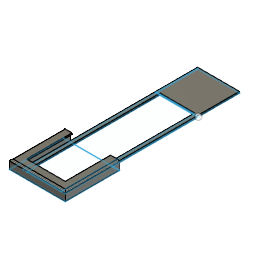
assembled (Autodesk Fusion 360 archive; units mm, degrees)
design "Dongle v3"
part number: 2026-08-27-20-51-44-399
Autodesk Fusion 360 part; units mm, degrees
sketch "snippy-Edge_Cuts" plane through (0, 0, 0) normal (0, 1, 0) x (1, 0, 0)
  line L0 (73.4, -145) -> (85.6, -145)
  line L1 (85.6, -145) -> (85.6, -157)
  line L2 (85.6, -157) -> (73.4, -157)
  line L3 (73.4, -157) -> (73.4, -145)
  line L4 (73.4, -145) -> (73.4, -157)
  line L5 (73.4, -157) -> (85.6, -157)
  line L6 (85.6, -157) -> (85.6, -195.7)
  line L7 (85.6, -195.7) -> (73.4, -195.7)
  line L8 (73.4, -195.7) -> (73.4, -157)
  line L9 (87.6, -182) -> (87.6, -197.7)
  line L10 (87.6, -197.7) -> (71.4, -197.7)
  line L11 (71.4, -197.7) -> (71.4, -182)
  line L12 (73.4, -157) -> (85.6, -157)
  line L13 (84.5, -157) -> (74.5, -157)
  line L14 (74.5, -157) -> (74.5, -195.7)
  line L15 (74.5, -195.7) -> (84.5, -195.7)
  line L16 (84.5, -195.7) -> (84.5, -157)
  line L17 (85.6, -157) -> (85.6, -182)
  line L18 (85.6, -182) -> (87.6, -182)
  line L19 (87.6, -182) -> (71.4, -182)
  dimension "d4" = 12
  dimension "d8" = 12.2
  dimension "d9" = 12.2
  dimension "d23" = 10
  dimension "d25" = 1.1
  dimension "d26" = 1.1
  constraint horizontal L0
  constraint vertical L1
  constraint horizontal L2
  constraint vertical L3
  constraint perpendicular L2 L4
  constraint horizontal L5
  constraint vertical L6
  constraint horizontal L7
  constraint vertical L8
  constraint perpendicular L1 L12
  constraint horizontal L13
  constraint vertical L14
  constraint horizontal L15
  constraint vertical L16
  constraint coincident L7 L14.end
  constraint coincident L2 L13.start
  constraint vertical L17
  constraint horizontal L18
  constraint perpendicular L11 L19
  measures "d4" distance of L0.start L2.end
  measures "d8" distance of L0.start L0.end
  measures "d9" distance of L6.end L7.end
  measures "d23" distance of L13.start L13.end
  measures "d25" distance of L1.end L13.start
  measures "d26" distance of L2.end L13.end
extrude "Extrude6" add sketch "snippy-Edge_Cuts" along normal blind 0.4 contours L0 L1 L2 L3 L4 L5 L12 L13 | L2 L5 L8 L12 L14 L19 | L2 L5 L6 L12 L16 L17 L19 | L7 L8 L14 L19 | L6 L7 L8 L9 L10 L11 L15 L18 L19 | L6 L7 L16 L19 makes body 1
extrude "Extrude7" cut sketch "snippy-Edge_Cuts" along normal blind 2.6 contours L6 L7 L8 L9 L10 L11 L15 L18 L19 bodies 1
extrude "Extrude8" add sketch "snippy-Edge_Cuts" along normal blind 2.2 contours L6 L7 L8 L9 L10 L11 L15 L18 L19 bodies 1
extrude "Extrude9" add 1 faces at (77.4667, 2.2, 197.0333) along direction (0, 1, 0) blind 0.4 separate body on bodies 1 makes body 2
sketch "Sketch6" plane through (0, 2.6, 0) normal (0, 1, 0) x (-1, 0, 0)
  line L0 (-87.6, 197.7) -> (-87.6, 182)
  line L1 (-87.6, 182) -> (-85.6, 182)
  line L2 (-85.6, 182) -> (-85.6, 195.7)
  line L3 (-85.6, 195.7) -> (-73.4, 195.7)
  line L4 (-73.4, 195.7) -> (-73.4, 182)
  line L5 (-73.4, 182) -> (-71.4, 182)
  line L6 (-71.4, 182) -> (-71.4, 197.7)
  line L7 (-71.4, 197.7) -> (-87.6, 197.7)
  line L8 (-85.1, 182) -> (-85.1, 195.2)
  line L9 (-85.1, 195.2) -> (-73.9, 195.2)
  line L10 (-73.9, 195.2) -> (-73.9, 182)
  line L11 (-85.1, 182) -> (-85.6, 182)
  line L12 (-85.6, 182) -> (-85.6, 195.7)
  line L13 (-85.6, 195.7) -> (-73.4, 195.7)
  line L14 (-73.4, 195.7) -> (-73.4, 182)
  line L15 (-73.4, 182) -> (-73.9, 182)
  dimension "d40" = 0.5
  constraint coincident L1.end L2.start
  constraint perpendicular L2 L11
  constraint coincident L2.end L3.start
  constraint coincident L3.end L4.start
  constraint coincident L4.end L5.start
  constraint perpendicular L10 L15
extrude "Extrude10" add sketch "Sketch6" against normal blind 0.4 contours L2 L3 L4 L8 L9 L10 L11 L12 L13 L14 L15 bodies 1 2
fillet "Fillet2" radius 0.5 3 edges at (87.6, 2.6, 189.85) (79.5, 2.6, 197.7) (71.4, 2.6, 189.85) on bodies 1
sketch "Sketch3" plane through (0, 2.6, 0) normal (0, 1, 0) x (-1, 0, 0)
  line L0 (-85.6, 195.7) -> (-85.6, 157)
  line L1 (-73.4, 195.7) -> (-85.6, 195.7)
  line L2 (-73.4, 157) -> (-73.4, 195.7)
  line L3 (-85.6, 157) -> (-73.4, 157)
  line L4 (-85.1, 195.7) -> (-85.6, 195.7)
  line L5 (-73.9, 157) -> (-85.6, 157)
  line L6 (-85.6, 157) -> (-73.4, 157)
  line L7 (-73.4, 157) -> (-73.4, 195.7)
  line L8 (-73.4, 195.7) -> (-85.6, 195.7)
  line L9 (-73.9, 157) -> (-73.9, 195.2)
  line L10 (-73.9, 195.2) -> (-85.1, 195.2)
  line L11 (-85.1, 195.2) -> (-85.1, 157)
  dimension "d17" = 0.5
  constraint coincident L0.start L1.end
  constraint perpendicular L0 L4
  constraint coincident L0.end L3.start
  constraint perpendicular L2 L5
  constraint coincident L2.start L3.end
  constraint coincident L1.start L2.end
sketch "Sketch4" plane through (0, 0.4, 0) normal (0, 1, 0) x (-1, 0, 0)
  line L0 (-73.4, 145) -> (-73.4, 195.7)
  line L1 (-85.6, 195.7) -> (-85.6, 145)
  line L2 (-85.6, 145) -> (-73.4, 145)
  line L3 (-73.4, 195.7) -> (-85.6, 195.7)
